Autodesk Inventor part; units mm, degrees
(part 5 of 5)
  line L168 (-15.0692, 74.0272) -> (-15.0692, 72.2893)
  spline S71 degree 2 poles (-15.0692, 72.2893) (-15.0692, 72.0854) (-14.9381, 71.9495) (-14.7464, 71.9495) knots 0 0 0 1 2 2 2
  line L169 (-14.7464, 71.9495) -> (-14.7002, 71.9495)
  line L170 (-14.7002, 71.9495) -> (-14.7002, 71.1)
  line L171 (-14.7002, 71.1) -> (-14.9308, 71.1)
  spline S72 degree 2 poles (-14.9308, 71.1) (-15.409, 71.1) (-15.9405, 71.6558) (-15.9405, 72.1485) knots 0 0 0 1 2 2 2
  line L172 (-15.9405, 72.1485) -> (-15.9405, 74.0272)
  spline S73 degree 2 poles (-13.0182, 74.1) (-12.3968, 74.1) (-11.5085, 73.1947) (-11.5085, 72.5636) knots 0 0 0 1 2 2 2
  spline S74 degree 2 poles (-11.5085, 72.5636) (-11.5085, 71.9228) (-12.4041, 71.0272) (-13.0449, 71.0272) knots 0 0 0 1 2 2 2
  spline S75 degree 2 poles (-13.0449, 71.0272) (-13.6808, 71.0272) (-14.5813, 71.9277) (-14.5813, 72.5636) knots 0 0 0 1 2 2 2
  spline S76 degree 2 poles (-14.5813, 72.5636) (-14.5813, 73.2068) (-13.676, 74.1) (-13.0182, 74.1) knots 0 0 0 1 2 2 2
  spline S77 degree 2 poles (-13.0449, 73.2383) (-13.3119, 73.2383) (-13.6905, 72.8427) (-13.6905, 72.566) knots 0 0 0 1 2 2 2
  spline S78 degree 2 poles (-13.6905, 72.566) (-13.6905, 72.2869) (-13.3119, 71.8913) (-13.0449, 71.8913) knots 0 0 0 1 2 2 2
  spline S79 degree 2 poles (-13.0449, 71.8913) (-12.7755, 71.8913) (-12.3993, 72.2845) (-12.3993, 72.566) knots 0 0 0 1 2 2 2
  spline S80 degree 2 poles (-12.3993, 72.566) (-12.3993, 72.8451) (-12.7755, 73.2383) (-13.0449, 73.2383) knots 0 0 0 1 2 2 2
  line L173 (-8.0595, 74.0272) -> (-8.0595, 71.9204)
  spline S81 degree 2 poles (-8.0595, 71.9204) (-8.0595, 71.5248) (-8.5352, 71.0272) (-8.9114, 71.0272) knots 0 0 0 1 2 2 2
  spline S82 degree 2 poles (-8.9114, 71.0272) (-9.3677, 71.0272) (-9.608, 71.4422) knots 0 0 0 1 1 1
  spline S83 degree 2 poles (-9.608, 71.4422) (-9.7561, 71.2189) (-10.0934, 71.0272) (-10.3434, 71.0272) knots 0 0 0 1 2 2 2
  spline S84 degree 2 poles (-10.3434, 71.0272) (-10.7391, 71.0272) (-11.159, 71.5248) (-11.159, 71.9932) knots 0 0 0 1 2 2 2
  line L174 (-11.159, 71.9932) -> (-11.159, 74.0272)
  line L175 (-11.159, 74.0272) -> (-10.2876, 74.0272)
  line L176 (-10.2876, 74.0272) -> (-10.2876, 72.1243)
  spline S85 degree 2 poles (-10.2876, 72.1243) (-10.2876, 71.9811) (-10.2415, 71.8913) (-10.1735, 71.8913) knots 0 0 0 1 2 2 2
  spline S86 degree 2 poles (-10.1735, 71.8913) (-10.0449, 71.8913) (-10.0449, 72.1073) knots 0 0 0 1 1 1
  line L177 (-10.0449, 72.1073) -> (-10.0449, 74.0272)
  line L178 (-10.0449, 74.0272) -> (-9.1735, 74.0272)
  line L179 (-9.1735, 74.0272) -> (-9.1735, 72.1243)
  spline S87 degree 2 poles (-9.1735, 72.1243) (-9.1735, 71.9859) (-9.1274, 71.8913) (-9.0595, 71.8913) knots 0 0 0 1 2 2 2
  spline S88 degree 2 poles (-9.0595, 71.8913) (-8.9308, 71.8913) (-8.9308, 72.1243) knots 0 0 0 1 1 1
  line L180 (-8.9308, 72.1243) -> (-8.9308, 74.0272)
  line L181 (-8.9308, 74.0272) -> (-8.0595, 74.0272)
  line L182 (-4.8273, 89.1874) -> (-4.8273, 87.1)
  line L183 (-4.8273, 87.1) -> (-5.6987, 87.1)
  line L184 (-5.6987, 87.1) -> (-5.6987, 90.0272)
  line L185 (-5.6987, 90.0272) -> (-4.5652, 90.0272)
  spline S89 degree 2 poles (-4.5652, 90.0272) (-3.8176, 90.0272) (-3.3977, 89.6874) knots 0 0 0 1 1 1
  spline S90 degree 2 poles (-3.3977, 89.6874) (-2.8953, 89.282) (-2.8953, 88.5879) knots 0 0 0 1 1 1
  spline S91 degree 2 poles (-2.8953, 88.5879) (-2.8953, 87.9228) (-3.7521, 87.083) (-4.4268, 87.083) knots 0 0 0 1 2 2 2
  spline S92 degree 2 poles (-4.4268, 87.083) (-4.5069, 87.083) (-4.6866, 87.0903) knots 0 0 0 1 1 1
  line L186 (-4.6866, 87.0903) -> (-4.6866, 87.9519)
  line L187 (-4.6866, 87.9519) -> (-4.5482, 87.9519)
  spline S93 degree 2 poles (-4.5482, 87.9519) (-3.7861, 87.9519) (-3.7861, 88.5879) knots 0 0 0 1 1 1
  spline S94 degree 2 poles (-3.7861, 88.5879) (-3.7861, 89.1874) (-4.5336, 89.1874) knots 0 0 0 1 1 1
  line L188 (-4.5336, 89.1874) -> (-4.8273, 89.1874)
  line L189 (-35.3847, 72.9811) -> (-35.3847, 72.2092)
  line L190 (-35.3847, 72.2092) -> (-35.625, 72.2092)
  line L191 (-35.625, 72.2092) -> (-35.625, 71.1)
  line L192 (-35.625, 71.1) -> (-36.4964, 71.1)
  line L193 (-36.4964, 71.1) -> (-36.4964, 74.0272)
  line L194 (-36.4964, 74.0272) -> (-35.625, 74.0272)
  line L195 (-35.625, 74.0272) -> (-35.625, 72.9811)
  line L196 (-35.625, 72.9811) -> (-35.3847, 72.9811)
  line L197 (-34.3653, 74.0272) -> (-34.3653, 71.1)
  line L198 (-34.3653, 71.1) -> (-35.2367, 71.1)
  line L199 (-35.2367, 71.1) -> (-35.2367, 74.0272)
  line L200 (-35.2367, 74.0272) -> (-34.3653, 74.0272)
  line L201 (-32.909, 74.0272) -> (-32.909, 71.1)
  line L202 (-32.909, 71.1) -> (-33.7803, 71.1)
  line L203 (-33.7803, 71.1) -> (-33.7803, 74.0272)
  line L204 (-33.7803, 74.0272) -> (-32.909, 74.0272)
  line L205 (-31.0837, 72.7408) -> (-30.2561, 72.7408)
  spline S95 degree 2 poles (-30.2561, 72.7408) (-29.9867, 72.4083) (-29.9867, 72.0393) knots 0 0 0 1 1 1
  spline S96 degree 2 poles (-29.9867, 72.0393) (-29.9867, 71.6097) (-30.6153, 71.0272) (-31.074, 71.0272) knots 0 0 0 1 2 2 2
  spline S97 degree 2 poles (-31.074, 71.0272) (-31.6687, 71.0272) (-32.5012, 71.9325) (-32.5012, 72.583) knots 0 0 0 1 2 2 2
  spline S98 degree 2 poles (-32.5012, 72.583) (-32.5012, 73.2335) (-31.6541, 74.1) (-31.0206, 74.1) knots 0 0 0 1 2 2 2
  spline S99 degree 2 poles (-31.0206, 74.1) (-30.8046, 74.1) (-30.54, 74.0126) knots 0 0 0 1 1 1
  line L206 (-30.54, 74.0126) -> (-30.54, 73.1413)
  spline S100 degree 2 poles (-30.54, 73.1413) (-30.7464, 73.2383) (-30.9163, 73.2383) knots 0 0 0 1 1 1
  spline S101 degree 2 poles (-30.9163, 73.2383) (-31.2221, 73.2383) (-31.6104, 72.8573) (-31.6104, 72.5515) knots 0 0 0 1 2 2 2
  spline S102 degree 2 poles (-31.6104, 72.5515) (-31.6104, 72.2408) (-31.2512, 71.8767) (-30.943, 71.8767) knots 0 0 0 1 2 2 2
  spline S103 degree 2 poles (-30.943, 71.8767) (-30.7488, 71.8767) (-30.7488, 71.9908) knots 0 0 0 1 1 1
  spline S104 degree 2 poles (-30.7488, 71.9908) (-30.7488, 72.0757) (-30.875, 72.0757) knots 0 0 0 1 1 1
  line L207 (-30.875, 72.0757) -> (-31.0837, 72.0757)
  line L208 (-31.0837, 72.0757) -> (-31.0837, 72.7408)
  line L209 (-28.5206, 72.9811) -> (-28.5206, 72.2092)
  line L210 (-28.5206, 72.2092) -> (-28.7609, 72.2092)
  line L211 (-28.7609, 72.2092) -> (-28.7609, 71.1)
  line L212 (-28.7609, 71.1) -> (-29.6323, 71.1)
  line L213 (-29.6323, 71.1) -> (-29.6323, 74.0272)
  line L214 (-29.6323, 74.0272) -> (-28.7609, 74.0272)
  line L215 (-28.7609, 74.0272) -> (-28.7609, 72.9811)
  line L216 (-28.7609, 72.9811) -> (-28.5206, 72.9811)
  line L217 (-27.5012, 74.0272) -> (-27.5012, 71.1)
  line L218 (-27.5012, 71.1) -> (-28.3726, 71.1)
  line L219 (-28.3726, 71.1) -> (-28.3726, 74.0272)
  line L220 (-28.3726, 74.0272) -> (-27.5012, 74.0272)
  spline S105 degree 2 poles (-23.3908, 77.0485) (-22.9765, 77.0485) (-22.3843, 76.445) (-22.3843, 76.0243) knots 0 0 0 1 2 2 2
  spline S106 degree 2 poles (-22.3843, 76.0243) (-22.3843, 75.5971) (-22.9814, 75) (-23.4086, 75) knots 0 0 0 1 2 2 2
  spline S107 degree 2 poles (-23.4086, 75) (-23.8325, 75) (-24.4328, 75.6003) (-24.4328, 76.0243) knots 0 0 0 1 2 2 2
  spline S108 degree 2 poles (-24.4328, 76.0243) (-24.4328, 76.4531) (-23.8293, 77.0485) (-23.3908, 77.0485) knots 0 0 0 1 2 2 2
  spline S109 degree 2 poles (-23.4086, 76.4741) (-23.5866, 76.4741) (-23.839, 76.2104) (-23.839, 76.0259) knots 0 0 0 1 2 2 2
  spline S110 degree 2 poles (-23.839, 76.0259) (-23.839, 75.8398) (-23.5866, 75.5761) (-23.4086, 75.5761) knots 0 0 0 1 2 2 2
  spline S111 degree 2 poles (-23.4086, 75.5761) (-23.229, 75.5761) (-22.9782, 75.8382) (-22.9782, 76.0259) knots 0 0 0 1 2 2 2
  spline S112 degree 2 poles (-22.9782, 76.0259) (-22.9782, 76.212) (-23.229, 76.4741) (-23.4086, 76.4741) knots 0 0 0 1 2 2 2
  line L221 (-21.3778, 76.0793) -> (-21.3778, 75.5566)
  line L222 (-21.3778, 75.5566) -> (-21.5704, 75.5566)
  line L223 (-21.5704, 75.5566) -> (-21.5704, 75.0485)
  line L224 (-21.5704, 75.0485) -> (-22.1513, 75.0485)
  line L225 (-22.1513, 75.0485) -> (-22.1513, 76.2589)
  spline S113 degree 2 poles (-22.1513, 76.2589) (-22.1513, 76.6003) (-21.729, 77.0485) (-21.4086, 77.0485) knots 0 0 0 1 2 2 2
  spline S114 degree 2 poles (-21.4086, 77.0485) (-21.0558, 77.0485) (-20.8196, 76.7443) knots 0 0 0 1 1 1
  line L226 (-20.8196, 76.7443) -> (-21.2953, 76.3964)
  spline S115 degree 2 poles (-21.2953, 76.3964) (-21.3341, 76.5081) (-21.4361, 76.5081) knots 0 0 0 1 1 1
  spline S116 degree 2 poles (-21.4361, 76.5081) (-21.5704, 76.5081) (-21.5704, 76.322) knots 0 0 0 1 1 1
  line L227 (-21.5704, 76.322) -> (-21.5704, 76.0793)
  line L228 (-21.5704, 76.0793) -> (-21.3778, 76.0793)
  line L229 (-19.9684, 76.0793) -> (-19.9684, 75.5566)
  line L230 (-19.9684, 75.5566) -> (-20.161, 75.5566)
  line L231 (-20.161, 75.5566) -> (-20.161, 75.0485)
  line L232 (-20.161, 75.0485) -> (-20.7419, 75.0485)
  line L233 (-20.7419, 75.0485) -> (-20.7419, 76.2589)
  spline S117 degree 2 poles (-20.7419, 76.2589) (-20.7419, 76.6003) (-20.3196, 77.0485) (-19.9992, 77.0485) knots 0 0 0 1 2 2 2
  spline S118 degree 2 poles (-19.9992, 77.0485) (-19.6464, 77.0485) (-19.4102, 76.7443) knots 0 0 0 1 1 1
  line L234 (-19.4102, 76.7443) -> (-19.8859, 76.3964)
  spline S119 degree 2 poles (-19.8859, 76.3964) (-19.9248, 76.5081) (-20.0267, 76.5081) knots 0 0 0 1 1 1
  spline S120 degree 2 poles (-20.0267, 76.5081) (-20.161, 76.5081) (-20.161, 76.322) knots 0 0 0 1 1 1
  line L235 (-20.161, 76.322) -> (-20.161, 76.0793)
  line L236 (-20.161, 76.0793) -> (-19.9684, 76.0793)
  spline S121 degree 2 poles (-22.8439, 63) (-22.4296, 63) (-21.8374, 62.3964) (-21.8374, 61.9757) knots 0 0 0 1 2 2 2
  spline S122 degree 2 poles (-21.8374, 61.9757) (-21.8374, 61.5485) (-22.4345, 60.9515) (-22.8617, 60.9515) knots 0 0 0 1 2 2 2
  spline S123 degree 2 poles (-22.8617, 60.9515) (-23.2856, 60.9515) (-23.8859, 61.5518) (-23.8859, 61.9757) knots 0 0 0 1 2 2 2
  spline S124 degree 2 poles (-23.8859, 61.9757) (-23.8859, 62.4045) (-23.2824, 63) (-22.8439, 63) knots 0 0 0 1 2 2 2
  spline S125 degree 2 poles (-22.8617, 62.4256) (-23.0396, 62.4256) (-23.2921, 62.1618) (-23.2921, 61.9773) knots 0 0 0 1 2 2 2
  spline S126 degree 2 poles (-23.2921, 61.9773) (-23.2921, 61.7913) (-23.0396, 61.5275) (-22.8617, 61.5275) knots 0 0 0 1 2 2 2
  spline S127 degree 2 poles (-22.8617, 61.5275) (-22.682, 61.5275) (-22.4312, 61.7896) (-22.4312, 61.9773) knots 0 0 0 1 2 2 2
  spline S128 degree 2 poles (-22.4312, 61.9773) (-22.4312, 62.1634) (-22.682, 62.4256) (-22.8617, 62.4256) knots 0 0 0 1 2 2 2
  line L237 (-21.6044, 61) -> (-21.6044, 62.267)
  spline S129 degree 2 poles (-21.6044, 62.267) (-21.6044, 62.6003) (-21.2047, 63) (-20.8746, 63) knots 0 0 0 1 2 2 2
  spline S130 degree 2 poles (-20.8746, 63) (-20.5429, 63) (-20.1934, 62.6117) (-20.1934, 62.2476) knots 0 0 0 1 2 2 2
  line L238 (-20.1934, 62.2476) -> (-20.1934, 61)
  line L239 (-20.1934, 61) -> (-20.7743, 61)
  line L240 (-20.7743, 61) -> (-20.7743, 62.2476)
  spline S131 degree 2 poles (-20.7743, 62.2476) (-20.7743, 62.4256) (-20.9005, 62.4256) knots 0 0 0 1 1 1
  spline S132 degree 2 poles (-20.9005, 62.4256) (-21.0235, 62.4256) (-21.0235, 62.2476) knots 0 0 0 1 1 1
  line L241 (-21.0235, 62.2476) -> (-21.0235, 61)
  line L242 (-21.0235, 61) -> (-21.6044, 61)
  spline S133 degree 2 poles (-42.8439, 63) (-42.4296, 63) (-41.8374, 62.3964) (-41.8374, 61.9757) knots 0 0 0 1 2 2 2
  spline S134 degree 2 poles (-41.8374, 61.9757) (-41.8374, 61.5485) (-42.4345, 60.9515) (-42.8617, 60.9515) knots 0 0 0 1 2 2 2
  spline S135 degree 2 poles (-42.8617, 60.9515) (-43.2856, 60.9515) (-43.8859, 61.5518) (-43.8859, 61.9757) knots 0 0 0 1 2 2 2
  spline S136 degree 2 poles (-43.8859, 61.9757) (-43.8859, 62.4045) (-43.2824, 63) (-42.8439, 63) knots 0 0 0 1 2 2 2
  spline S137 degree 2 poles (-42.8617, 62.4256) (-43.0396, 62.4256) (-43.2921, 62.1618) (-43.2921, 61.9773) knots 0 0 0 1 2 2 2
  spline S138 degree 2 poles (-43.2921, 61.9773) (-43.2921, 61.7913) (-43.0396, 61.5275) (-42.8617, 61.5275) knots 0 0 0 1 2 2 2
  spline S139 degree 2 poles (-42.8617, 61.5275) (-42.682, 61.5275) (-42.4312, 61.7896) (-42.4312, 61.9773) knots 0 0 0 1 2 2 2
  spline S140 degree 2 poles (-42.4312, 61.9773) (-42.4312, 62.1634) (-42.682, 62.4256) (-42.8617, 62.4256) knots 0 0 0 1 2 2 2
  line L243 (-41.6044, 61) -> (-41.6044, 62.267)
  spline S141 degree 2 poles (-41.6044, 62.267) (-41.6044, 62.6003) (-41.2047, 63) (-40.8746, 63) knots 0 0 0 1 2 2 2
  spline S142 degree 2 poles (-40.8746, 63) (-40.5429, 63) (-40.1934, 62.6117) (-40.1934, 62.2476) knots 0 0 0 1 2 2 2
  line L244 (-40.1934, 62.2476) -> (-40.1934, 61)
  line L245 (-40.1934, 61) -> (-40.7743, 61)
  line L246 (-40.7743, 61) -> (-40.7743, 62.2476)
  spline S143 degree 2 poles (-40.7743, 62.2476) (-40.7743, 62.4256) (-40.9005, 62.4256) knots 0 0 0 1 1 1
  spline S144 degree 2 poles (-40.9005, 62.4256) (-41.0235, 62.4256) (-41.0235, 62.2476) knots 0 0 0 1 1 1
  line L247 (-41.0235, 62.2476) -> (-41.0235, 61)
  line L248 (-41.0235, 61) -> (-41.6044, 61)
  spline S145 degree 2 poles (-43.3908, 77.0485) (-42.9765, 77.0485) (-42.3843, 76.445) (-42.3843, 76.0243) knots 0 0 0 1 2 2 2
  spline S146 degree 2 poles (-42.3843, 76.0243) (-42.3843, 75.5971) (-42.9814, 75) (-43.4086, 75) knots 0 0 0 1 2 2 2
  spline S147 degree 2 poles (-43.4086, 75) (-43.8325, 75) (-44.4328, 75.6003) (-44.4328, 76.0243) knots 0 0 0 1 2 2 2
  spline S148 degree 2 poles (-44.4328, 76.0243) (-44.4328, 76.4531) (-43.8293, 77.0485) (-43.3908, 77.0485) knots 0 0 0 1 2 2 2
  spline S149 degree 2 poles (-43.4086, 76.4741) (-43.5866, 76.4741) (-43.839, 76.2104) (-43.839, 76.0259) knots 0 0 0 1 2 2 2
  spline S150 degree 2 poles (-43.839, 76.0259) (-43.839, 75.8398) (-43.5866, 75.5761) (-43.4086, 75.5761) knots 0 0 0 1 2 2 2
  spline S151 degree 2 poles (-43.4086, 75.5761) (-43.229, 75.5761) (-42.9782, 75.8382) (-42.9782, 76.0259) knots 0 0 0 1 2 2 2
  spline S152 degree 2 poles (-42.9782, 76.0259) (-42.9782, 76.212) (-43.229, 76.4741) (-43.4086, 76.4741) knots 0 0 0 1 2 2 2
  line L249 (-41.3778, 76.0793) -> (-41.3778, 75.5566)
  line L250 (-41.3778, 75.5566) -> (-41.5704, 75.5566)
  line L251 (-41.5704, 75.5566) -> (-41.5704, 75.0485)
  line L252 (-41.5704, 75.0485) -> (-42.1513, 75.0485)
  line L253 (-42.1513, 75.0485) -> (-42.1513, 76.2589)
  spline S153 degree 2 poles (-42.1513, 76.2589) (-42.1513, 76.6003) (-41.729, 77.0485) (-41.4086, 77.0485) knots 0 0 0 1 2 2 2
  spline S154 degree 2 poles (-41.4086, 77.0485) (-41.0558, 77.0485) (-40.8196, 76.7443) knots 0 0 0 1 1 1
  line L254 (-40.8196, 76.7443) -> (-41.2953, 76.3964)
  spline S155 degree 2 poles (-41.2953, 76.3964) (-41.3341, 76.5081) (-41.4361, 76.5081) knots 0 0 0 1 1 1
  spline S156 degree 2 poles (-41.4361, 76.5081) (-41.5704, 76.5081) (-41.5704, 76.322) knots 0 0 0 1 1 1
  line L255 (-41.5704, 76.322) -> (-41.5704, 76.0793)
  line L256 (-41.5704, 76.0793) -> (-41.3778, 76.0793)
  line L257 (-39.9684, 76.0793) -> (-39.9684, 75.5566)
  line L258 (-39.9684, 75.5566) -> (-40.161, 75.5566)
  line L259 (-40.161, 75.5566) -> (-40.161, 75.0485)
  line L260 (-40.161, 75.0485) -> (-40.7419, 75.0485)
  line L261 (-40.7419, 75.0485) -> (-40.7419, 76.2589)
  spline S157 degree 2 poles (-40.7419, 76.2589) (-40.7419, 76.6003) (-40.3196, 77.0485) (-39.9992, 77.0485) knots 0 0 0 1 2 2 2
  spline S158 degree 2 poles (-39.9992, 77.0485) (-39.6464, 77.0485) (-39.4102, 76.7443) knots 0 0 0 1 1 1
  line L262 (-39.4102, 76.7443) -> (-39.8859, 76.3964)
  spline S159 degree 2 poles (-39.8859, 76.3964) (-39.9248, 76.5081) (-40.0267, 76.5081) knots 0 0 0 1 1 1
  spline S160 degree 2 poles (-40.0267, 76.5081) (-40.161, 76.5081) (-40.161, 76.322) knots 0 0 0 1 1 1
  line L263 (-40.161, 76.322) -> (-40.161, 76.0793)
  line L264 (-40.161, 76.0793) -> (-39.9684, 76.0793)
  line L265 (-12.3358, 79) -> (-11.7549, 79)
  line L266 (-11.7549, 79) -> (-11.7549, 77.8414)
  spline S161 degree 2 poles (-11.7549, 77.8414) (-11.7549, 77.7055) (-11.6675, 77.6149) (-11.5396, 77.6149) knots 0 0 0 1 2 2 2
  line L267 (-11.5396, 77.6149) -> (-11.5089, 77.6149)
  line L268 (-11.5089, 77.6149) -> (-11.5089, 77.0485)
  line L269 (-11.5089, 77.0485) -> (-11.6626, 77.0485)
  spline S162 degree 2 poles (-11.6626, 77.0485) (-11.9814, 77.0485) (-12.3358, 77.4191) (-12.3358, 77.7476) knots 0 0 0 1 2 2 2
  line L270 (-12.3358, 77.7476) -> (-12.3358, 79)
  line L271 (-11.7759, 92.0307) -> (-11.7759, 91.5081)
  line L272 (-11.7759, 91.5081) -> (-11.9684, 91.5081)
  line L273 (-11.9684, 91.5081) -> (-11.9684, 91)
  line L274 (-11.9684, 91) -> (-12.5494, 91)
  line L275 (-12.5494, 91) -> (-12.5494, 92.2104)
  spline S163 degree 2 poles (-12.5494, 92.2104) (-12.5494, 92.5518) (-12.127, 93) (-11.8066, 93) knots 0 0 0 1 2 2 2
  spline S164 degree 2 poles (-11.8066, 93) (-11.4539, 93) (-11.2176, 92.6958) knots 0 0 0 1 1 1
  line L276 (-11.2176, 92.6958) -> (-11.6934, 92.3479)
  spline S165 degree 2 poles (-11.6934, 92.3479) (-11.7322, 92.4595) (-11.8341, 92.4595) knots 0 0 0 1 1 1
  spline S166 degree 2 poles (-11.8341, 92.4595) (-11.9684, 92.4595) (-11.9684, 92.2735) knots 0 0 0 1 1 1
  line L277 (-11.9684, 92.2735) -> (-11.9684, 92.0307)
  line L278 (-11.9684, 92.0307) -> (-11.7759, 92.0307)
  line L279 (-31.9684, 92.254) -> (-31.9684, 91.7395)
  line L280 (-31.9684, 91.7395) -> (-32.1286, 91.7395)
  line L281 (-32.1286, 91.7395) -> (-32.1286, 91)
  line L282 (-32.1286, 91) -> (-32.7095, 91)
  line L283 (-32.7095, 91) -> (-32.7095, 92.9515)
  line L284 (-32.7095, 92.9515) -> (-32.1286, 92.9515)
  line L285 (-32.1286, 92.9515) -> (-32.1286, 92.254)
  line L286 (-32.1286, 92.254) -> (-31.9684, 92.254)
  line L287 (-31.2888, 92.9515) -> (-31.2888, 91)
  line L288 (-31.2888, 91) -> (-31.8697, 91)
  line L289 (-31.8697, 91) -> (-31.8697, 92.9515)
  line L290 (-31.8697, 92.9515) -> (-31.2888, 92.9515)
  line L291 (-31.4935, 78.9595) -> (-31.4935, 78.4045)
  spline S167 degree 2 poles (-31.4935, 78.4045) (-31.5566, 78.4256) (-31.5906, 78.4256) knots 0 0 0 1 1 1
  spline S168 degree 2 poles (-31.5906, 78.4256) (-31.657, 78.4256) (-31.7508, 78.3285) (-31.7508, 78.2605) knots 0 0 0 1 2 2 2
  spline S169 degree 2 poles (-31.7508, 78.2605) (-31.7508, 78.2006) (-31.699, 78.1117) knots 0 0 0 1 1 1
  line L292 (-31.699, 78.1117) -> (-31.6553, 78.034)
  spline S170 degree 2 poles (-31.6553, 78.034) (-31.5356, 77.8252) (-31.5356, 77.6311) knots 0 0 0 1 1 1
  spline S171 degree 2 poles (-31.5356, 77.6311) (-31.5356, 77.3463) (-31.9401, 76.9515) (-32.2314, 76.9515) knots 0 0 0 1 2 2 2
  spline S172 degree 2 poles (-32.2314, 76.9515) (-32.3706, 76.9515) (-32.5081, 77.0162) knots 0 0 0 1 1 1
  line L293 (-32.5081, 77.0162) -> (-32.5081, 77.5809)
  spline S173 degree 2 poles (-32.5081, 77.5809) (-32.4256, 77.5275) (-32.3608, 77.5275) knots 0 0 0 1 1 1
  spline S174 degree 2 poles (-32.3608, 77.5275) (-32.2864, 77.5275) (-32.1845, 77.6149) (-32.1845, 77.6812) knots 0 0 0 1 2 2 2
  spline S175 degree 2 poles (-32.1845, 77.6812) (-32.1845, 77.7233) (-32.2654, 77.8673) knots 0 0 0 1 1 1
  spline S176 degree 2 poles (-32.2654, 77.8673) (-32.3948, 78.0971) (-32.3948, 78.3252) knots 0 0 0 1 1 1
  spline S177 degree 2 poles (-32.3948, 78.3252) (-32.3948, 78.6019) (-32.0016, 79) (-31.7298, 79) knots 0 0 0 1 2 2 2
  spline S178 degree 2 poles (-31.7298, 79) (-31.6084, 79) (-31.4935, 78.9595) knots 0 0 0 1 1 1
  point P0 (0, 0)
  point P1 (-22, 90.1)
  point P2 (-2, 90.1)
  point P3 (-32, 74.1)
  point P4 (-12, 74.1)
  point P5 (0, 82.6286)
  point P6 (0, 89.2497)
  point P7 (-22, 63)
  point P8 (-22, 78.6821)
  point P9 (-42, 79.3847)
  point P10 (-42, 63)
  point P11 (-32, 94.9889)
  point P12 (-12, 97.0363)
  point P13 (-32, 79)
  point P14 (-12, 79)
  point P15 (-32, 91)
  point P16 (-12, 91)
  point P17 (-42, 75)
  point P18 (-22, 75)
  dimension "d136" = 10
  dimension "d137" = 10
  dimension "d138" = 10
  dimension "d139" = 10
  dimension "d140" = 10
  dimension "d141" = 6
  dimension "d142" = 6
  dimension "d143" = 6
  dimension "d144" = 6
  dimension "d145" = 6
  dimension "d146" = 6
  dimension "d147" = 6
  dimension "d148" = 6
  constraints: 24 tangent, 19 midpoint, 6 end point, 2 parallel, 2 vertical, 1 perpendicular, 30 other
  measures "d136" distance of L12.start L12.end
  measures "d137" horizontal distance of point (-22, 90.1) A3.centre
  measures "d138" horizontal distance of point (-2, 90.1) A4.centre
  measures "d139" horizontal distance of point (-32, 74.1) A5.centre
  measures "d140" horizontal distance of point (-12, 74.1) A6.centre
  measures "d141" distance of A3.centre point (-32, 91)
  measures "d142" distance of point (-32, 79) A3.centre
  measures "d143" distance of A4.centre point (-12, 91)
  measures "d144" distance of point (-12, 79) A4.centre
  measures "d145" distance of point (-42, 75) A5.centre
  measures "d146" distance of point (-42, 63) A5.centre
  measures "d147" distance of point (-22, 75) A6.centre
  measures "d148" distance of point (-22, 63) A6.centre
extrude "Wyciągnięcie proste16" add sketch "Szkic19" along normal up to surface (0.6 mm away) contours L64 L65 S0 L66 L67 L68 S1 L69 | L70 L71 S2 S3 L72 L73 L74 S4 L75 S5 L76 L77 L78 S6 S7 L79 | L80 L81 L82 L83 L84 L85 | L86 L87 S8 S9 L88 L89 L90 S10 L91 S11 L92 L93 L94 S12 S13 L95 | L96 L97 S14 L98 L99 L100 S15 L101 | L102 S16 S17 S18 S19 S20 L103 S21 S22 S23 S24 S25 L104 L105 | L106 L107 L108 L109 L110 S26 S27 L111 L112 L113 S28 S29 L114 L115 | L116 L117 L118 L119 | L120 S30 S31 L121 L122 L123 S32 S33 L124 L125 | L126 L127 L128 L129 L130 L131 L132 L133 | S34 S35 S36 S37 | L134 S42 S43 L135 L136 L137 S44 S45 L138 L139 | L140 L141 S46 S47 L142 L143 L144 S48 L145 S49 L146 L147 L148 S50 S51 L149 | L150 S52 S53 S54 S55 S56 L151 S57 S58 S59 S60 | L152 L153 S61 L154 L155 L156 S62 L157 | L158 L159 L160 L161 | L162 S63 S64 S65 L163 L164 L165 S66 S67 S68 S69 S70 L166 | L167 L168 S71 L169 L170 L171 S72 L172 | S73 S74 S75 S76 | L173 S81 S82 S83 S84 L174 L175 L176 S85 S86 L177 L178 L179 S87 S88 L180 L181 | L182 L183 L184 L185 S89 S90 S91 S92 L186 L187 S93 S94 L188 | L189 L190 L191 L192 L193 L194 L195 L196 | L197 L198 L199 L200 | L201 L202 L203 L204 | L205 S95 S96 S97 S98 S99 L206 S100 S101 S102 S103 S104 L207 L208 | L209 L210 L211 L212 L213 L214 L215 L216 | L217 L218 L219 L220 | S105 S106 S107 S108 | L221 L222 L223 L224 L225 S113 S114 L226 S115 S116 L227 L228 | L229 L230 L231 L232 L233 S117 S118 L234 S119 S120 L235 L236 | S121 S122 S123 S124 | L237 S129 S130 L238 L239 L240 S131 S132 L241 L242 | S133 S134 S135 S136 | L243 S141 S142 L244 L245 L246 S143 S144 L247 L248 | S145 S146 S147 S148 | L249 L250 L251 L252 L253 S153 S154 L254 S155 S156 L255 L256 | L257 L258 L259 L260 L261 S157 S158 L262 S159 S160 L263 L264 | L265 L266 S161 L267 L268 L269 S162 L270 | L271 L272 L273 L274 L275 S163 S164 L276 S165 S166 L277 L278 | L279 L280 L281 L282 L283 L284 L285 L286 | L287 L288 L289 L290 | L291 S167 S168 S169 L292 S170 S171 S172 L293 S173 S174 S175 S176 S177 S178
equation "\"d0\" = obudowa_a"
equation "\"d1\" = obudowa_b"
equation "\"d2\" = obudowa_wys"
equation "\"d4\" = obudowa_grubosc"
equation "\"d6\" = obudowa_wys"
equation "\"d16\" = obudowa_otwory_montazowe_material_x"
equation "\"d17\" = obudowa_otwory_montazowe_material_y"
equation "\"d20\" = obudowa_otwory_montazowe_poz_x"
equation "\"d21\" = obudowa_otwory_montazowe_poz_y"
equation "\"d22\" = insert_D"
equation "\"d24\" = gniazdo_M2_D1"
equation "\"d25\" = gniazdo_M2_glebokosc"
equation "\"d27\" = insert_glebokosc"
equation "\"d29\" = obudowa_zaokraglenie"
equation "\"d30\" = obudowa_otwory_io1_wys"
equation "\"d39\" = obudowa_otwory_io1_poz"
equation "\"d32\" = obudowa_otwory_io1_D"
equation "\"d37\" = insert_glebokosc"
equation "\"d40\" = obudowa_otwory_io2_wys"
equation "\"d41\" = obudowa_otwory_io2_poz"
equation "\"d42\" = obudowa_otwory_io2_D"
equation "\"d62\" = obudowa_otwory_pot_D"
equation "\"d65\" = obudowa_pot_poz_x"
equation "\"d66\" = obudowa_pot_poz_y"
equation "\"d67\" = obudowa_pot_rozstaw"
equation "\"d69\" = obudowa_s_rozstaw_y"
equation "\"d70\" = obudowa_s_D"
equation "\"d71\" = obudowa_s_rozstaw_x"
equation "\"d54\" = input_wys"
equation "\"d55\" = input_a"
equation "\"obudowa_podkladka_otwory\" = 4"
equation "\"gniazdo_M2_glebokosc\" = 1.5"
equation "\"gniazdo_M2_D1\" = 4.5"
equation "\"gniazdo_M2_D2\" = 2.6"
equation "\"podstawa_wys\" = 2"
equation "\"podstawa_otwory_montazowe_poz_x\" = 4"
equation "\"podstawa_otwory_montazowe_poz_y\" = 4"
equation "\"obudowa_b\" = 110"
equation "\"obudowa_a\" = 100"
equation "\"obudowa_wys\" = 45"
equation "\"obudowa_grubosc\" = 2"
equation "\"d5\" = -obudowa_grubosc"
equation "\"obudowa_prowadnica_odsuniecie\" = 2"
equation "\"obudowa_prowadnica_grubosc\" = 2"
equation "\"obudowa_kontrolki_a\" = 38"
equation "\"obudowa_prowadnica_wys\" = 19"
equation "\"obudowa_otwory_montazowe_poz_y\" = 4"
equation "\"obudowa_otwory_montazowe_poz_x\" = 4"
equation "\"obudowa_otwory_montazowe_material_y\" = 8"
equation "\"obudowa_otwory_montazowe_material_x\" = 8"
equation "\"insert_D\" = 2.4"
equation "\"insert_glebokosc\" = 5.5"
equation "\"obudowa_zaokraglenie\" = 3"
equation "\"podstawa_zaokraglenie\" = 3"
equation "\"obudowa_otwory_io_wys\" = 15"
equation "\"obudowa_otwory_io_D\" = 15"
equation "\"obudowa_otwory_io1_poz\" = 55"
equation "\"obudowa_otwory_io1_wys\" = 25"
equation "\"obudowa_otwory_io1_D\" = 11.5"
equation "\"obudowa_otwory_io2_poz\" = 38"
equation "\"obudowa_otwory_io2_wys\" = 25"
equation "\"obudowa_otwory_io2_D\" = 11.5"
equation "\"obudowa_otwory_pot_D\" = 8"
equation "\"input_b\" = 14.4"
equation "\"input_wys\" = 11"
equation "\"input_a\" = 9"
equation "\"obudowa_MTS_otwor_D\" = 6.2"
equation "\"obudowa_pot_rozstaw\" = 30"
equation "\"obudowa_pot_poz_y\" = 15"
equation "\"obudowa_pot_poz_x\" = 20"
equation "\"obudowa_s_poz_x\" = 78"
equation "\"obudowa_s_D\" = 6.2"
equation "\"obudowa_s_poz_y\" = 15"
equation "\"obudowa_s_rozstaw_x\" = 10"
equation "\"obudowa_s_rozstaw_y\" = 16"
equation "\"pcb_rozstaw_x\" = 92"
equation "\"pcb_rozstaw_y\" = 58"
equation "\"obudowa_pcb_grubosc_scianki\" = 6"
equation "\"pcb_grubosc_scianki\" = 6"
equation "\"pcb_poz_y\" = 27"
equation "\"pcb_wys_bloku\" = 35"
equation "\"obudowa_footswitch_poz_y\" = 68"
equation "\"obudowa_footswitch_poz_x\" = 35"
equation "\"obudowa_footswitch_D\" = 12.3"
equation "\"obudowa_led_indicator_D\" = 4"
equation "\"obudowa_led_indicator_poz_x\" = 55"
